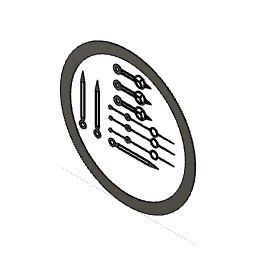
Hands (Autodesk Fusion 360 design; units mm, degrees)
Autodesk Fusion 360 part; units mm, degrees
sketch "Sketch1" plane through (0, 0, 0) normal (0, 0, 1) x (1, 0, 0)
  circle A0 centre (0, 0) radius 14.986
  constraint coincident A0.centre origin
sketch "Sketch2" plane through (0, 0, 0) normal (0, 0, 1) x (1, 0, 0)
  line L0 (0, 0) -> (5.1345, 0)
  line L1 (5.1345, 0) -> (-12.3806, 0)
  constraint coincident L0.start origin
  constraint horizontal L0
  constraint parallel L0 L1
sketch "Sketch3" plane through (0, 0, 0) normal (0, 0, 1) x (1, 0, 0)
  line L0 (-8.1021, 0.0936) -> (-11.5779, 0.0936)
  circle A0 centre (-0.3485, 0) radius 0.7451
  line L1 (-8.1021, -0.0945) -> (-11.5779, -0.0945)
  line L2 (-6.7019, 0.0936) -> (-1.348, 0.0936)
  line L3 (0.6509, 0.0936) -> (2.9828, 0.0936)
  line L4 (-6.7019, -0.0945) -> (-1.3479, -0.0945)
  line L5 (0.6508, -0.0945) -> (2.9828, -0.0945)
  arc A1 (-1.3479, -0.0945) -> (0.6508, -0.0945) centre (-0.3485, 0) ccw
  arc A2 (0.6509, 0.0936) -> (-1.348, 0.0936) centre (-0.3485, 0) ccw
  arc A3 (-11.5779, 0.0936) -> (-11.5779, -0.0945) centre (-12.0115, -0.0005) ccw
  arc A4 (-8.1021, -0.0945) -> (-6.7019, -0.0945) centre (-7.402, -0.0005) ccw
  arc A5 (-6.7019, 0.0936) -> (-8.1021, 0.0936) centre (-7.402, -0.0005) ccw
  line L6 (5.1064, -0.0005) -> (2.9828, 0.0936)
  line L7 (2.9828, -0.0945) -> (5.1064, -0.0005)
  circle A6 centre (-10.2492, 12.2135) radius 0.4287
  line L8 (-9.3449, 12.7329) -> (-5.5698, 12.7329)
  line L9 (-9.236, 12.4605) -> (-5.6455, 12.4605)
  line L10 (-2.8889, 12.7329) -> (-1.1611, 12.2135)
  line L11 (-2.8154, 12.4732) -> (-1.7969, 12.2135)
  arc A7 (-2.8889, 12.7329) -> (-5.5698, 12.7329) centre (-4.2293, 12.2135) ccw
  line L12 (-9.3449, 11.6942) -> (-5.5698, 11.6942)
  line L13 (-9.236, 11.9665) -> (-5.6455, 11.9665)
  arc A8 (-5.5698, 11.6942) -> (-2.8889, 11.6942) centre (-4.2293, 12.2135) ccw
  line L14 (-2.8889, 11.6942) -> (-1.1611, 12.2135)
  line L15 (-2.8154, 11.9538) -> (-1.7969, 12.2135)
  arc A9 (-9.3449, 12.7329) -> (-9.3449, 11.6942) centre (-10.2492, 12.2135) ccw
  arc A10 (-9.236, 11.9665) -> (-9.236, 12.4605) centre (-10.2492, 12.2135) ccw
  arc A11 (-5.6455, 12.4605) -> (-5.6455, 11.9665) centre (-4.2293, 12.2135) ccw
  arc A12 (-5.5698, 11.6942) -> (-2.8889, 11.6942) centre (-4.2293, 12.2135) ccw
  arc A13 (-2.8154, 11.9538) -> (-2.8154, 12.4732) centre (-4.2293, 12.2135) ccw
  line L16 (-4.2293, 12.2135) -> (-3.0608, 12.2135) construction
  line L17 (-4.2825, 12.3274) -> (-5.3923, 12.3274)
  line L18 (-3.9372, 12.7195) -> (-4.0264, 12.771)
  line L19 (-4.0264, 12.771) -> (-4.2825, 12.3274)
  line L20 (-4.0264, 12.771) -> (-3.7366, 13.273)
  line L21 (-3.8492, 11.7583) -> (-3.5593, 11.2562)
  line L22 (-3.8492, 11.7583) -> (-4.1041, 12.2244)
  line L23 (-3.848, 12.668) -> (-4.1041, 12.2244)
  line L24 (-3.848, 12.668) -> (-3.5581, 13.17)
  line L25 (-4.2922, 12.0997) -> (-3.7353, 11.1546)
  line L26 (-4.8136, 12.0997) -> (-5.3923, 12.0997)
  line L27 (-4.8136, 12.0997) -> (-4.2922, 12.0997)
  line L28 (-4.2825, 12.3274) -> (-3.7366, 13.273)
  arc A14 (-3.7366, 13.273) -> (-5.3923, 12.3274) centre (-4.2293, 12.2135) ccw
  arc A15 (-5.3923, 12.0997) -> (-3.7353, 11.1546) centre (-4.2293, 12.2135) ccw
  arc A16 (-3.5593, 11.2562) -> (-3.5581, 13.17) centre (-4.2293, 12.2135) ccw
  circle A17 centre (-15.6062, -5.4607) radius 0.4523
  line L29 (-16.1225, 4.3796) -> (-15.6062, 6.9994)
  line L30 (-16.1225, 4.3796) -> (-16.1225, -3.7992)
  line L31 (-16.1225, -3.7992) -> (-15.8643, -4.6162)
  line L32 (-15.0898, -3.7992) -> (-15.348, -4.6162)
  line L33 (-15.0898, 4.3796) -> (-15.0898, -3.7992)
  line L34 (-15.0898, 4.3796) -> (-15.6062, 6.9994)
  line L35 (-15.296, 0.2902) -> (-15.296, 4.3796)
  line L36 (-15.9163, -3.7992) -> (-15.296, -3.7992)
  line L37 (-15.296, 0.2902) -> (-15.296, -3.7992)
  line L38 (-15.9163, 0.2902) -> (-15.9163, 4.3796)
  line L39 (-15.9163, 0.2902) -> (-15.9163, -3.7992)
  arc A18 (-15.8643, -4.6162) -> (-15.348, -4.6162) centre (-15.6062, -5.4607) ccw
  line L40 (-15.9163, 4.3796) -> (-15.296, 4.3796)
  circle A19 centre (-7.402, -0.0005) radius 0.1568
  circle A20 centre (-7.402, -0.0005) radius 15.4432
  circle A21 centre (-7.402, -0.0005) radius 18.0594
  circle A22 centre (-10.2009, 8.546) radius 0.4287
  arc A23 (-2.7672, 8.2863) -> (-2.7672, 8.8057) centre (-4.1811, 8.546) ccw
  line L41 (-3.7997, 9.0005) -> (-4.0559, 8.5568)
  line L42 (-3.801, 8.0908) -> (-3.511, 7.5887)
  line L43 (-3.9782, 9.1035) -> (-3.6883, 9.6055)
  line L44 (-9.2966, 8.0267) -> (-5.5215, 8.0267)
  line L45 (-9.1878, 8.793) -> (-5.5972, 8.793)
  arc A24 (-2.8406, 9.0653) -> (-5.5215, 9.0653) centre (-4.1811, 8.546) ccw
  arc A25 (-5.5215, 8.0267) -> (-2.8406, 8.0267) centre (-4.1811, 8.546) ccw
  arc A26 (-5.344, 8.4321) -> (-3.687, 7.4871) centre (-4.1811, 8.546) ccw
  line L46 (-9.2966, 9.0653) -> (-5.5215, 9.0653)
  line L47 (-3.8889, 9.052) -> (-3.9782, 9.1035)
  line L48 (-4.2343, 8.6599) -> (-5.344, 8.6599)
  arc A27 (-3.511, 7.5887) -> (-3.5099, 9.5025) centre (-4.1811, 8.546) ccw
  line L49 (-4.2343, 8.6599) -> (-3.6883, 9.6055)
  line L50 (-3.801, 8.0908) -> (-4.0559, 8.5568)
  line L51 (-4.7653, 8.4321) -> (-5.344, 8.4321)
  line L52 (-4.1811, 8.546) -> (-3.0126, 8.546) construction
  arc A28 (-9.2966, 9.0653) -> (-9.2966, 8.0267) centre (-10.2009, 8.546) ccw
  arc A29 (-9.1878, 8.299) -> (-9.1878, 8.793) centre (-10.2009, 8.546) ccw
  line L53 (-3.9782, 9.1035) -> (-4.2343, 8.6599)
  line L54 (-9.1878, 8.299) -> (-5.5972, 8.299)
  arc A30 (-5.5972, 8.793) -> (-5.5972, 8.299) centre (-4.1811, 8.546) ccw
  arc A31 (-5.5215, 8.0267) -> (-2.8406, 8.0267) centre (-4.1811, 8.546) ccw
  arc A32 (-3.6883, 9.6055) -> (-5.344, 8.6599) centre (-4.1811, 8.546) ccw
  line L55 (-2.8406, 9.0653) -> (-1.1129, 8.546)
  line L56 (-4.7653, 8.4321) -> (-4.2439, 8.4321)
  line L57 (-2.7672, 8.2863) -> (-1.7486, 8.546)
  line L58 (-4.2439, 8.4321) -> (-3.687, 7.4871)
  line L59 (-2.7672, 8.8057) -> (-1.7486, 8.546)
  line L60 (-2.8406, 8.0267) -> (-1.1129, 8.546)
  line L61 (-3.7997, 9.0005) -> (-3.5099, 9.5025)
  circle A33 centre (-10.1044, 4.975) radius 0.4287
  arc A34 (-2.6706, 4.7153) -> (-2.6706, 5.2347) centre (-4.0846, 4.975) ccw
  line L62 (-3.7032, 5.4295) -> (-3.9593, 4.9858)
  line L63 (-3.7044, 4.5198) -> (-3.4145, 4.0177)
  line L64 (-3.8817, 5.5325) -> (-3.5918, 6.0345)
  line L65 (-9.2001, 4.4557) -> (-5.425, 4.4557)
  line L66 (-9.0913, 5.222) -> (-5.5007, 5.222)
  arc A35 (-2.7441, 5.4943) -> (-5.425, 5.4943) centre (-4.0846, 4.975) ccw
  arc A36 (-5.425, 4.4557) -> (-2.7441, 4.4557) centre (-4.0846, 4.975) ccw
  arc A37 (-5.2475, 4.8611) -> (-3.5905, 3.9161) centre (-4.0846, 4.975) ccw
  line L67 (-9.2001, 5.4943) -> (-5.425, 5.4943)
  line L68 (-3.7924, 5.481) -> (-3.8817, 5.5325)
  line L69 (-4.1378, 5.0889) -> (-5.2475, 5.0889)
  arc A38 (-3.4145, 4.0177) -> (-3.4134, 5.9315) centre (-4.0846, 4.975) ccw
  line L70 (-4.1378, 5.0889) -> (-3.5918, 6.0345)
  line L71 (-3.7044, 4.5198) -> (-3.9593, 4.9858)
  line L72 (-4.6688, 4.8611) -> (-5.2475, 4.8611)
  line L73 (-4.0846, 4.975) -> (-2.916, 4.975) construction
  arc A39 (-9.2001, 5.4943) -> (-9.2001, 4.4557) centre (-10.1044, 4.975) ccw
  arc A40 (-9.0913, 4.728) -> (-9.0913, 5.222) centre (-10.1044, 4.975) ccw
  line L74 (-3.8817, 5.5325) -> (-4.1378, 5.0889)
  line L75 (-9.0913, 4.728) -> (-5.5007, 4.728)
  arc A41 (-5.5007, 5.222) -> (-5.5007, 4.728) centre (-4.0846, 4.975) ccw
  arc A42 (-5.425, 4.4557) -> (-2.7441, 4.4557) centre (-4.0846, 4.975) ccw
  arc A43 (-3.5918, 6.0345) -> (-5.2475, 5.0889) centre (-4.0846, 4.975) ccw
  line L76 (-2.7441, 5.4943) -> (-1.0164, 4.975)
  line L77 (-4.6688, 4.8611) -> (-4.1474, 4.8611)
  line L78 (-2.6706, 4.7153) -> (-1.6521, 4.975)
  line L79 (-4.1474, 4.8611) -> (-3.5905, 3.9161)
  line L80 (-2.6706, 5.2347) -> (-1.6521, 4.975)
  line L81 (-2.7441, 4.4557) -> (-1.0164, 4.975)
  line L82 (-3.7032, 5.4295) -> (-3.4134, 5.9315)
  arc A44 (-19.7731, -4.4232) -> (-19.2568, -4.4232) centre (-19.515, -5.2677) ccw
  line L83 (-19.8251, -3.6062) -> (-19.2048, -3.6062)
  line L84 (-18.9986, -3.6062) -> (-19.2568, -4.4232)
  circle A45 centre (-19.515, -5.2677) radius 0.4523
  line L85 (-20.0313, -3.6062) -> (-19.7731, -4.4232)
  line L86 (-19.8251, 0.4832) -> (-19.8251, -3.6062)
  line L87 (-20.0313, 4.5726) -> (-20.0313, -3.6062)
  line L88 (-19.2048, 0.4832) -> (-19.2048, 4.5726)
  line L89 (-18.9986, 4.5726) -> (-18.9986, -3.6062)
  line L90 (-19.2048, 0.4832) -> (-19.2048, -3.6062)
  line L91 (-19.8251, 4.5726) -> (-19.2048, 4.5726)
  line L92 (-18.9986, 4.5726) -> (-19.515, 7.1924)
  line L93 (-20.0313, 4.5726) -> (-19.515, 7.1924)
  line L94 (-19.8251, 0.4832) -> (-19.8251, 4.5726)
  line L95 (5.0098, 2.4606) -> (2.8863, 2.5547)
  arc A46 (-1.4444, 2.3666) -> (0.5543, 2.3666) centre (-0.4451, 2.4611) ccw
  line L96 (-8.1987, 2.5547) -> (-11.6744, 2.5547)
  arc A47 (-11.6744, 2.5547) -> (-11.6744, 2.3666) centre (-12.108, 2.4606) ccw
  arc A48 (-8.1987, 2.3666) -> (-6.7984, 2.3666) centre (-7.4985, 2.4606) ccw
  line L97 (-8.1987, 2.3666) -> (-11.6744, 2.3666)
  line L98 (0.5544, 2.5547) -> (2.8863, 2.5547)
  circle A49 centre (-7.4985, 2.4606) radius 0.1568
  circle A50 centre (-0.4451, 2.4611) radius 0.7451
  line L99 (2.8863, 2.3666) -> (5.0098, 2.4606)
  arc A51 (0.5544, 2.5547) -> (-1.4445, 2.5547) centre (-0.4451, 2.4611) ccw
  line L100 (0.5543, 2.3666) -> (2.8863, 2.3666)
  line L101 (-6.7984, 2.5547) -> (-1.4445, 2.5547)
  line L102 (-6.7984, 2.3666) -> (-1.4444, 2.3666)
  arc A52 (-6.7984, 2.5547) -> (-8.1987, 2.5547) centre (-7.4985, 2.4606) ccw
  line L103 (5.0098, -2.7994) -> (2.8863, -2.7053)
  arc A53 (-1.4444, -2.8934) -> (0.5543, -2.8934) centre (-0.4451, -2.7989) ccw
  line L104 (-8.1987, -2.7053) -> (-11.6744, -2.7053)
  arc A54 (-11.6744, -2.7053) -> (-11.6744, -2.8934) centre (-12.108, -2.7994) ccw
  arc A55 (-8.1987, -2.8934) -> (-6.7984, -2.8934) centre (-7.4985, -2.7994) ccw
  line L105 (-8.1987, -2.8934) -> (-11.6744, -2.8934)
  line L106 (0.5544, -2.7053) -> (2.8863, -2.7053)
  circle A56 centre (-7.4985, -2.7994) radius 0.1568
  circle A57 centre (-0.4451, -2.7989) radius 0.7451
  line L107 (2.8863, -2.8934) -> (5.0098, -2.7994)
  arc A58 (0.5544, -2.7053) -> (-1.4445, -2.7053) centre (-0.4451, -2.7989) ccw
  line L108 (0.5543, -2.8934) -> (2.8863, -2.8934)
  line L109 (-6.7984, -2.7053) -> (-1.4445, -2.7053)
  line L110 (-6.7984, -2.8934) -> (-1.4444, -2.8934)
  arc A59 (-6.7984, -2.7053) -> (-8.1987, -2.7053) centre (-7.4985, -2.7994) ccw
  circle A60 centre (-11.6422, -5.4606) radius 0.4523
  line L111 (-5.8913, -5.7707) -> (-9.9807, -5.7707)
  line L112 (-9.9807, -4.9442) -> (-10.7977, -5.2024)
  line L113 (-1.8019, -4.9442) -> (-9.9807, -4.9442)
  line L114 (-1.8019, -5.9769) -> (0.8179, -5.4606)
  line L115 (-5.8913, -5.1504) -> (-1.8019, -5.1504)
  line L116 (-1.8019, -4.9442) -> (0.8179, -5.4606)
  line L117 (-1.8019, -5.9769) -> (-9.9807, -5.9769)
  line L118 (-5.8913, -5.7707) -> (-1.8019, -5.7707)
  line L119 (-1.8019, -5.1504) -> (-1.8019, -5.7707)
  line L120 (-9.9807, -5.9769) -> (-10.7977, -5.7187)
  line L121 (-9.9807, -5.1504) -> (-9.9807, -5.7707)
  line L122 (-5.8913, -5.1504) -> (-9.9807, -5.1504)
  arc A61 (-10.7977, -5.2024) -> (-10.7977, -5.7187) centre (-11.6422, -5.4606) ccw
  point P0 (-7.4985, 2.4606)
  point P1 (-7.4985, 2.4606)
  point P2 (-0.0965, 2.4611)
  point P3 (-7.4985, -2.7994)
  point P4 (-7.4985, -2.7994)
  point P5 (-0.0965, -2.7989)
  constraint horizontal L0
  constraint horizontal L2
  constraint concentric A0 A1
  constraint collinear L2 L3
  constraint collinear L4 L5
  constraint concentric A1 A2
  constraint concentric A4 A5
  constraint concentric A6 A9
  constraint concentric A7 A14
  constraint coincident L9.end A7
  constraint concentric A7 A11
  constraint concentric A9 A10
  constraint concentric A11 A12
  constraint concentric A12 A13
  constraint horizontal L16
  constraint coincident A7.centre A8.centre
  constraint perpendicular L18 L19
  constraint perpendicular L18 L20
  constraint coincident L21.end A14
  constraint horizontal L27
  constraint concentric A14 A15
  constraint concentric A15 A16
  constraint concentric A17 A18
  constraint perpendicular L33 L36
  constraint perpendicular L36 L37
  constraint perpendicular L35 L40
  constraint concentric A4 A19
  constraint concentric A19 A20
  constraint concentric A4 A21
  constraint concentric A22 A28
  constraint concentric A24 A32
  constraint coincident L45.end A24
  constraint concentric A24 A30
  constraint concentric A28 A29
  constraint concentric A30 A31
  constraint concentric A23 A31
  constraint horizontal L52
  constraint coincident A23.centre A24.centre
  constraint perpendicular L47 L53
  constraint perpendicular L43 L47
  constraint coincident L42.end A32
  constraint horizontal L56
  constraint concentric A26 A32
  constraint concentric A26 A27
  constraint concentric A33 A39
  constraint concentric A35 A43
  constraint coincident L66.end A35
  constraint concentric A35 A41
  constraint concentric A39 A40
  constraint concentric A41 A42
  constraint concentric A34 A42
  constraint horizontal L73
  constraint coincident A34.centre A35.centre
  constraint perpendicular L68 L74
  constraint perpendicular L64 L68
  constraint coincident L63.end A43
  constraint horizontal L77
  constraint concentric A37 A43
  constraint concentric A37 A38
  constraint concentric A44 A45
  constraint perpendicular L83 L89
  constraint perpendicular L83 L90
  constraint perpendicular L88 L91
  constraint horizontal L96
  constraint horizontal L101
  constraint concentric A46 A50
  constraint collinear L98 L101
  constraint collinear L100 L102
  constraint concentric A46 A51
  constraint concentric A48 A52
  constraint concentric A48 A49
  constraint horizontal L104
  constraint horizontal L109
  constraint concentric A53 A57
  constraint collinear L106 L109
  constraint collinear L108 L110
  constraint concentric A53 A58
  constraint concentric A55 A59
  constraint concentric A55 A56
  constraint concentric A60 A61
  constraint perpendicular L117 L121
  constraint perpendicular L111 L121
  constraint perpendicular L118 L119
extrude "Extrude1" add sketch "Sketch3" along normal blind 0.127 makes body 1 at (-8.0502, 11.7849, 0) makes body 2 at (-11.9116, 0.0107, 0) makes body 3 at (-15.6062, 5.2529, 0) makes body 4 at (9.6606, -1.6649, 0) makes body 5 at (-8.002, 8.9746, 0) makes body 6 at (-7.9055, 5.4036, 0.127) makes body 7 at (-12.2226, -2.7255, 0) makes body 8 at (-0.9287, -5.4606, 0) makes body 9 at (-12.2226, 2.5345, 0) makes body 10 at (-19.515, 5.4459, 0)
